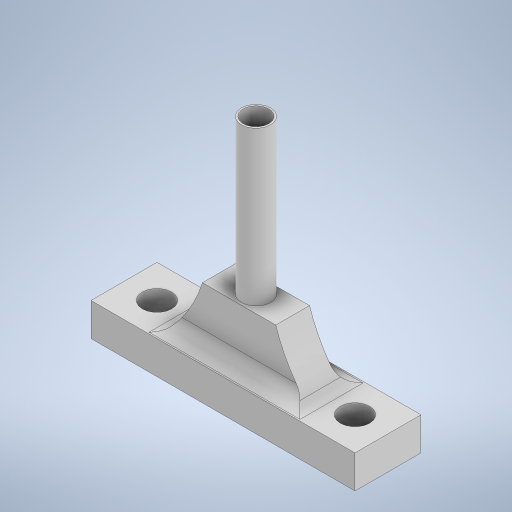
# Autodesk Inventor part: HUDSON-1-12 LEAFSPING SOLID EQUALISER
Saved by Autodesk Inventor 2024.2 (Build 282272000, 272)
## iProperties
Created: 2024-10-08
Part Number: HUDSON-1-12 LEAFSPING SOLID EQUALISER
Material: Generic
Document SubType Name: Modeling
Designer: Jimena Brenes
Density: 1 g/cm^3
Appearance: Default
Author: Jimena Brenes
Autodesk Inventor part; units mm, degrees
ref_plane "YZ Plane" through (0, 0, 0) normal (1, 0, 0) x (0, 1, 0)
ref_plane "XZ Plane" through (0, 0, 0) normal (0, 1, 0) x (-1, 0, 0)
ref_plane "XY Plane" through (0, 0, 0) normal (0, 0, 1) x (1, 0, 0)
sketch "Sketch1" plane through (0, 0, 0) normal (0, 0, 1) x (1, 0, 0)
  line L0 (0, 114) -> (0, -114) construction
  line L1 (-9.4, 0) -> (9.4, 0)
  line L2 (-5, 7.5) -> (5, 7.5)
  arc A0 (-9.4, 0) -> (-5, 7.5) centre (-24.038, 13.6283) ccw
  arc A1 (5, 7.5) -> (9.4, 0) centre (24.038, 13.6283) ccw
  point P0 (0, 0)
  point P1 (0, 0)
  point P2 (0, 7.5)
  dimension "d9" = 18.8
  dimension "d10" = 10
  dimension "d11" = 7.5
  dimension "d13" = 20
  constraints: 6 end point, 4 point on circle, 3 midpoint, 2 centre point, 2 horizontal, 1 coincident, 1 point on line, 1 symmetric about line, 1 vertical, 1 other
  measures "d9" distance of L1.start L1.end
  measures "d10" distance of L2.start L2.end
  measures "d11" distance between parallel lines of L1 L2
  measures "d13" radius of A0
extrude "Extrusion1" add sketch "Sketch1" along normal blind 4.6
sketch "Sketch2" plane through (-9.4, 0, 0) normal (0, -1, 0) x (1, 0, 0)
  line L0 (-8.6, 6.8) -> (27.4, 6.8)
  line L1 (27.4, 6.8) -> (27.4, -2.2)
  line L2 (27.4, -2.2) -> (-8.6, -2.2)
  line L3 (-8.6, -2.2) -> (-8.6, 6.8)
  line L4 (0, 4.6) -> (18.8, 4.6) projected
  line L5 (0, 0) -> (18.8, 0) projected
  line L6 (0, 0) -> (0, 4.6) projected
  line L7 (18.8, 0) -> (18.8, 4.6) projected
  point P0 (9.4, 0)
  point P1 (0, 2.3)
  dimension "d16" = 36
  dimension "d17" = 9
  dimension "d18" = 2.2
  dimension "d19" = 2.2
  dimension "d20" = 8.6
  dimension "d21" = 8.6
  constraints: 8 end point, 2 parallel, 1 horizontal, 1 midpoint, 1 perpendicular
  measures "d16" distance between parallel lines of L1 L3
  measures "d17" distance between parallel lines of L2 L0
  measures "d18" distance between parallel lines of L4 L0
  measures "d19" distance between parallel lines of L5 L2
  measures "d20" distance from line of point (0, 2.3) L3
  measures "d21" distance between parallel lines of L1 L7
extrude "Extrusion2" add sketch "Sketch2" along normal blind 4.5 contours L0 L1 L2 L3 | L4 L7 L5 L6
fillet "Fillet1" radius 2 4 edges at (0, 0, 4.6) (9.4, 0, 2.3) (0, 0, 0) (-9.4, 0, 2.3)
sketch "Sketch3" plane through (-5, 7.5, 0) normal (0, 1, 0) x (1, 0, 0)
  circle A0 centre (5, -2.3) radius 2
  circle A1 centre (5, -2.3) radius 1.75
  line L0 (10, -4.6) -> (0, -4.6) projected
  line L1 (10, 0) -> (0, 0) projected
  line L2 (0, 0) -> (0, -4.6) projected
  point P0 (5, 0)
  dimension "d25" = 4
  dimension "d26" = 3.5
  dimension "d27" = 2.3
  dimension "d28" = 2.3
  dimension "d29" = 5
  constraints: 2 centre point, 1 coincident
  measures "d25" diameter of A0
  measures "d26" diameter of A1
  measures "d27" distance from line of L0 A0.centre
  measures "d28" distance from line of L1 A0.centre
  measures "d29" distance from line of L2 A0.centre
extrude "Extrusion3" add sketch "Sketch3" along normal blind 21
sketch "Sketch4" plane through (-9.4, 0, 0) normal (0, 1, 0) x (1, 0, 0)
  circle A0 centre (-4.1, -2.3) radius 2
  circle A1 centre (22.9, -2.3) radius 2
  line L0 (-8.6, 2.2) -> (27.4, 2.2) projected
  circle A2 centre (9.4, -2.3) radius 1.75 projected
  circle A3 centre (9.4, -2.3) radius 2 projected
  circle A4 centre (9.4, -2.3) radius 1.75 projected
  circle A5 centre (9.4, -2.3) radius 1.75
  point P0 (9.4, 0)
  dimension "d32" = 4
  dimension "d33" = 4
  dimension "d34" = 4.5
  dimension "d35" = 4.5
  dimension "d36" = 3.5
  dimension "d37" = 13.5
  dimension "d38" = 13.5
  constraints: 3 centre point, 1 coincident
  measures "d32" diameter of A0
  measures "d33" diameter of A1
  measures "d34" distance from line of L0 A0.centre
  measures "d35" distance from line of L0 A1.centre
  measures "d36" diameter of A5
  measures "d37" distance of A2.centre A0.centre
  measures "d38" distance of A2.centre A1.centre
hole "Hole1" at (-13.5, 0, 2.3) at (13.5, 0, 2.3) direction (0, -1, 0) diameter 4 end through all
equation "\"d38\" = d37"
body "Solid1"
